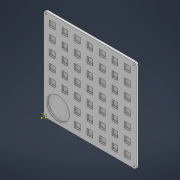
# Autodesk Inventor part: plade til cuvetter
Saved by Autodesk Inventor 2022 (Build 260153000, 153)
## iProperties
Created: 2022-06-14
Part Number: plade til cuvetter
Material: Generic
Document SubType Name: Modeling
Designer: Jakob Saugbjerg
Density: 1 g/cm^3
Appearance: Default
Author: Jakob Saugbjerg
Autodesk Inventor part; units mm, degrees
ref_plane "YZ Plane" through (0, 0, 0) normal (1, 0, 0) x (0, 1, 0)
ref_plane "XZ Plane" through (0, 0, 0) normal (0, 1, 0) x (-1, 0, 0)
ref_plane "XY Plane" through (0, 0, 0) normal (0, 0, 1) x (1, 0, 0)
sketch "Sketch1" plane through (0, 0, 0) normal (0, 0, 1) x (1, 0, 0)
  line L0 (0, 0) -> (220, 0)
  line L1 (220, 0) -> (220, 220)
  line L2 (220, 220) -> (0, 220)
  line L3 (0, 220) -> (0, 0)
  dimension "d0" = 220
  dimension "d1" = 220
  constraints: 8 end point, 2 parallel, 1 horizontal, 1 perpendicular
  measures "d0" distance of L2.end L1.end
  measures "d1" distance of L1.end L0.end
extrude "Extrusion1" add sketch "Sketch1" along normal blind 5
sketch "Sketch2" plane through (0, 0, 5) normal (0, 0, 1) x (1, 0, 0)
  line L0 (10, 210) -> (210, 210)
  line L1 (210, 210) -> (210, 10)
  line L2 (210, 10) -> (10, 10)
  line L3 (10, 10) -> (10, 210)
  line L4 (10, 210) -> (210, 10) construction
  line L5 (210, 210) -> (10, 10) construction
  line L6 (10, 210) -> (38.5, 210)
  line L7 (38.5, 210) -> (38.5, 181.5)
  line L8 (38.5, 181.5) -> (10, 181.5)
  line L9 (10, 181.5) -> (10, 210)
  circle A0 centre (24.25, 195.75) radius 10.25
  line L10 (17.75, 189.25) -> (30.75, 189.25)
  line L11 (30.75, 189.25) -> (30.75, 202.25)
  line L12 (30.75, 202.25) -> (17.75, 202.25)
  line L13 (17.75, 202.25) -> (17.75, 189.25)
  line L14 (17.75, 189.25) -> (30.75, 202.25) construction
  line L15 (30.75, 189.25) -> (17.75, 202.25) construction
  point P0 (0, 0)
  point P1 (110, 110)
  dimension "d4" = 200
  dimension "d5" = 200
  dimension "d6" = 28.5
  dimension "d7" = 28.5
  dimension "d8" = 20.5
  dimension "d41" = 13
  dimension "d42" = 13
  constraints: 32 end point, 6 parallel, 4 midpoint, 3 horizontal, 3 perpendicular, 1 centre point, 1 point on line
  measures "d4" distance of L1.end L2.end
  measures "d5" distance of L0.end L1.end
  measures "d6" distance of L7.end L8.end
  measures "d7" distance of L6.end L7.end
  measures "d8" diameter of A0
  measures "d41" distance of L12.end L11.end
  measures "d42" distance of L11.end L10.end
extrude "Extrusion2" cut sketch "Sketch2" against normal blind 3 contours L13 L12 L11 L10
pattern_linear "Rectangular Pattern1" count 7 spacing 28.5 along (1, 0, 0) count 5 spacing 28.5 along (0, -1, 0) of "Extrusion2"
sketch "Sketch4" plane through (0, 0, 5) normal (0, 0, 1) x (1, 0, 0)
  line L0 (210, 10) -> (10, 10)
  line L1 (10, 10) -> (10, 210)
  line L2 (10, 210) -> (210, 210)
  line L3 (210, 210) -> (210, 10)
  line L4 (210, 10) -> (10, 210) construction
  line L5 (10, 10) -> (210, 210) construction
  circle A0 centre (81.25, 81.75) radius 10.25 projected
  line L6 (81.25, 81.75) -> (81.25, 53.25)
  circle A1 centre (81.25, 53.25) radius 10.25
  line L7 (74.75, 46.75) -> (87.75, 46.75)
  line L8 (87.75, 46.75) -> (87.75, 59.75)
  line L9 (87.75, 59.75) -> (74.75, 59.75)
  line L10 (74.75, 59.75) -> (74.75, 46.75)
  line L11 (74.75, 46.75) -> (87.75, 59.75) construction
  line L12 (87.75, 46.75) -> (74.75, 59.75) construction
  point P0 (0, 0)
  point P1 (110, 110)
  dimension "d24" = 200
  dimension "d25" = 200
  dimension "d26" = 28.5
  dimension "d27" = 20.5
  dimension "d43" = 13
  dimension "d44" = 13
  constraints: 26 end point, 4 midpoint, 4 parallel, 2 horizontal, 2 perpendicular, 1 centre point, 1 coincident, 1 vertical
  measures "d24" distance of L1.end L2.end
  measures "d25" distance of L0.end L1.end
  measures "d26" distance of L6.start L6.end
  measures "d27" diameter of A1
  measures "d43" distance of L9.end L8.end
  measures "d44" distance of L8.end L7.end
extrude "Extrusion4" cut sketch "Sketch4" against normal blind 3 contours L9 L8 L7 L10
pattern_linear "Rectangular Pattern2" count 2 spacing 28.5 along (0, -1, 0) count 5 spacing 28.5 along (1, 0, 0) of "Extrusion4"
sketch "Sketch5" plane through (0, 0, 5) normal (0, 0, 1) x (1, 0, 0)
  line L0 (0, 0) -> (220, 0) projected
  line L1 (0, 0) -> (0, 5)
  line L2 (0, 220) -> (0, 0) projected
  line L3 (0, 5) -> (5, 5)
  circle A0 centre (5, 5) radius 1.6
  line L4 (220, 220) -> (0, 220) projected
  line L5 (110, 220) -> (110, 0)
  line L6 (220, 0) -> (220, 220) projected
  line L7 (220, 110) -> (0, 110)
  circle A1 centre (215, 5) radius 1.6
  circle A2 centre (5, 215) radius 1.6
  circle A3 centre (215, 215) radius 1.6
  dimension "d36" = 5
  dimension "d37" = 5
  dimension "d38" = 3.2
  constraints: 8 end point, 4 centre point, 4 midpoint, 3 symmetric about line, 1 coincident, 1 horizontal, 1 point on line, 3 other
  measures "d36" distance of L0.start L1.end
  measures "d37" distance of L1.end L3.end
  measures "d38" diameter of A0
extrude "Extrusion5" [suppressed]
sketch "Sketch6" plane through (0, 0, 5) normal (0, 0, 1) x (1, 0, 0)
  point P0 (0, 0)
sketch "Sketch3" plane through (0, 0, 5) normal (0, 0, 1) x (1, 0, 0)
  line L0 (10, 10) -> (210, 10)
  line L1 (210, 10) -> (210, 210)
  line L2 (210, 210) -> (10, 210)
  line L3 (10, 210) -> (10, 10)
  line L4 (10, 10) -> (210, 210) construction
  line L5 (210, 10) -> (10, 210) construction
  line L6 (10, 10) -> (65, 10)
  line L7 (65, 10) -> (65, 65)
  line L8 (65, 65) -> (10, 65)
  line L9 (10, 65) -> (10, 10)
  circle A0 centre (37.5, 37.5) radius 25.5
  point P0 (0, 0)
  point P1 (110, 110)
  dimension "d17" = 200
  dimension "d18" = 200
  dimension "d19" = 55
  dimension "d20" = 55
  dimension "d21" = 51
  constraints: 20 end point, 4 parallel, 2 horizontal, 2 midpoint, 2 perpendicular, 1 centre point, 1 point on line
  measures "d17" distance of L2.end L1.end
  measures "d18" distance of L1.end L0.end
  measures "d19" distance of L8.end L7.end
  measures "d20" distance of L7.end L6.end
  measures "d21" diameter of A0
extrude "Extrusion3" cut sketch "Sketch3" against normal blind 3 contours A0
fillet "Fillet1" radius 2 4 edges at (0, 220, 2.5) (220, 220, 2.5) (220, 0, 2.5) (0, 0, 2.5)
sketch "Sketch15" plane through (0, 0, 5) normal (0, 0, 1) x (1, 0, 0)
  line L0 (0, 0) -> (220, 0)
  line L1 (220, 0) -> (220, 220)
  line L2 (220, 220) -> (0, 220)
  line L3 (0, 220) -> (0, 0)
  line L4 (5, 5) -> (215, 5)
  line L5 (215, 5) -> (215, 215)
  line L6 (215, 215) -> (5, 215)
  line L7 (5, 215) -> (5, 5)
  line L8 (5, 5) -> (215, 215) construction
  line L9 (215, 5) -> (5, 215) construction
  line L10 (10, 10) -> (210, 10)
  line L11 (210, 10) -> (210, 210)
  line L12 (210, 210) -> (10, 210)
  line L13 (10, 210) -> (10, 10)
  line L14 (10, 10) -> (210, 210) construction
  line L15 (210, 10) -> (10, 210) construction
  circle A0 centre (10, 210) radius 1.75
  circle A1 centre (210, 210) radius 1.75
  circle A2 centre (10, 10) radius 1.75
  circle A3 centre (210, 10) radius 1.75
  point P0 (110, 110)
  dimension "d79" = 220
  dimension "d80" = 220
  dimension "d81" = 210
  dimension "d82" = 210
  dimension "d85" = 200
  dimension "d86" = 200
  dimension "d87" = 3.5
  dimension "d90" = 200
  dimension "d93" = 200
  constraints: 32 end point, 6 parallel, 4 centre point, 4 horizontal, 4 midpoint, 3 perpendicular, 1 coincident, 1 vertical, 6 other
  measures "d79" distance of L2.end L1.end
  measures "d80" distance of L1.end L0.end
  measures "d81" distance of L6.end L5.end
  measures "d82" distance of L5.end L4.end
  measures "d85" distance of L12.end L11.end
  measures "d86" distance of L11.end L10.end
  measures "d87" diameter of A0
  measures "d90" distance of A0.centre A1.centre
  measures "d93" distance of A0.centre A2.centre
extrude "Extrusion12" cut sketch "Sketch15" against normal blind 5 contours L3 L2 L1 L0 | L13 A2 L10 | L10 A2 L13 | A3 L11 L10 | L10 L11 A3 | A0 L12 L13 | L13 L12 A0 | A1 L12 L11 | L11 L12 A1
fillet "Fillet4" radius 4 4 edges at (5, 5, 2.5) (215, 5, 2.5) (215, 215, 2.5) (5, 215, 2.5)
sketch "Sketch16" plane through (0, 0, 5) normal (0, 0, 1) x (1, 0, 0)
  point P0 (5, 9)
  point P1 (9, 5)
body "Solid1"
